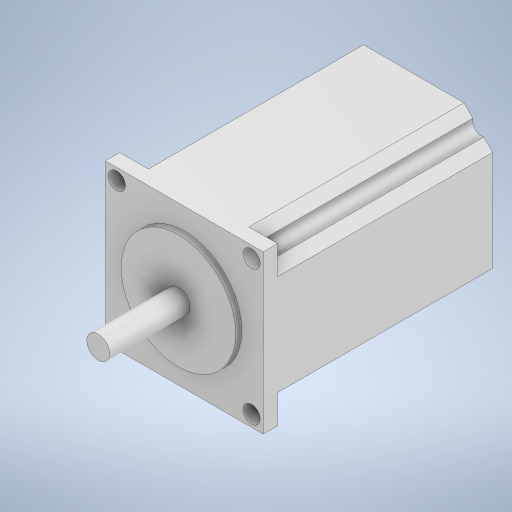
# Autodesk Inventor part: stepper motor base
Saved by Autodesk Inventor 2024 (Build 280153000, 153)
## iProperties
Created: 2023-10-26
Part Number: stepper motor base
Material: Aluminum
Document SubType Name: Modeling
Designer: mb
Density: 2.7 g/cm^3
Appearance: Satin
Author: mb
Autodesk Inventor part; units mm, degrees
ref_plane "YZ Plane" through (0, 0, 0) normal (1, 0, 0) x (0, 1, 0)
ref_plane "XZ Plane" through (0, 0, 0) normal (0, 1, 0) x (-1, 0, 0)
ref_plane "XY Plane" through (0, 0, 0) normal (0, 0, 1) x (1, 0, 0)
sketch "Sketch1" plane through (0, 0, 0) normal (0, 0, 1) x (1, 0, 0)
  line L0 (0, 0) -> (55, 0)
  line L1 (55, 0) -> (55, 55)
  line L2 (55, 55) -> (0, 55)
  line L3 (0, 55) -> (0, 0)
  dimension "d0" = 55
  dimension "d1" = 55
  constraints: 8 end point, 2 parallel, 1 horizontal, 1 perpendicular
  measures "d0" distance of L1.end L2.end
  measures "d1" distance of L0.end L1.end
extrude "Extrusion1" add sketch "Sketch1" along normal blind 80
sketch "Sketch2" plane through (0, 0, 80) normal (0, 0, 1) x (1, 0, 0)
  line L0 (55, 0) -> (55, 55) projected
  line L1 (55, 55) -> (0, 55) projected
  line L2 (0, 55) -> (0, 0) projected
  line L3 (0, 0) -> (55, 0) projected
  circle A0 centre (27.5, 27.5) radius 20
  circle A1 centre (27.5, 27.5) radius 4
  dimension "d7" = 27.5
  dimension "d8" = 27.5
  dimension "d9" = 40
  dimension "d10" = 8
  constraints: 2 centre point, 1 coincident
  measures "d7" distance from line of L1 A0.centre
  measures "d8" distance from line of L2 A0.centre
  measures "d9" diameter of A0
  measures "d10" diameter of A1
extrude "Extrusion2" add sketch "Sketch2" along normal blind 2 contours A0
sketch "Sketch3" plane through (27.5, 27.5, 80) normal (0, 0, 1) x (1, 0, 0)
  circle A0 centre (0, 0) radius 4 projected
  point P0 (-27.5, -27.5)
extrude "Extrusion3" add sketch "Sketch3" along normal blind 30
chamfer "Chamfer1" distance 10 angle 45 4 edges at (0, 55, 40) (0, 0, 40) (55, 0, 40) (55, 55, 40)
sketch "Sketch4" plane through (0, 0, 80) normal (0, 0, 1) x (1, 0, 0)
  line L0 (45, 55) -> (55, 45) projected
  line L1 (45, 55) -> (10, 55) projected
  line L2 (0, 45) -> (10, 55) projected
  line L3 (0, 45) -> (0, 10) projected
  line L4 (10, 0) -> (0, 10) projected
  line L5 (10, 0) -> (45, 0) projected
  line L6 (55, 10) -> (45, 0) projected
  line L7 (55, 10) -> (55, 45) projected
  circle A0 centre (27.5, 27.5) radius 20 projected
  line L8 (10, 55) -> (0, 55)
  line L9 (0, 55) -> (0, 45)
  line L10 (0, 10) -> (0, 0)
  line L11 (0, 0) -> (10, 0)
  line L12 (45, 0) -> (55, 0)
  line L13 (55, 0) -> (55, 10)
  line L14 (55, 45) -> (55, 55)
  line L15 (45, 55) -> (55, 55)
  constraints: 16 end point, 4 perpendicular, 4 point on line, 1 horizontal, 1 vertical
extrude "Extrusion4" add sketch "Sketch4" against normal blind 5 contours L15 L14 L0 | L2 L9 L8 | L13 L12 L6 | L4 L11 L10
sketch "Sketch5" plane through (0, 0, 80) normal (0, 0, 1) x (1, 0, 0)
  line L0 (0, 45) -> (10, 55) projected
  circle A0 centre (4, 51) radius 3
  line L1 (55, 55) -> (0, 55) projected
  line L2 (0, 55) -> (0, 0) projected
  circle A1 centre (4, 4) radius 3
  circle A2 centre (51, 4) radius 3
  circle A3 centre (51, 51) radius 3
  line L3 (0, 0) -> (55, 0) projected
  line L4 (55, 0) -> (55, 55) projected
  dimension "d20" = 4
  dimension "d21" = 4
  dimension "d22" = 6
  dimension "d23" = 4
  dimension "d24" = 4
  dimension "d25" = 4
  dimension "d26" = 4
  dimension "d27" = 4
  dimension "d28" = 4
  constraints: 4 centre point, 3 equal radius
  measures "d20" distance from line of L1 A0.centre
  measures "d21" distance from line of L2 A0.centre
  measures "d22" diameter of A0
  measures "d23" distance from line of L3 A1.centre
  measures "d24" distance from line of L2 A1.centre
  measures "d25" distance from line of L3 A2.centre
  measures "d26" distance from line of L4 A2.centre
  measures "d27" distance from line of L4 A3.centre
  measures "d28" distance from line of L1 A3.centre
extrude "Extrusion5" cut sketch "Sketch5" against normal through all contours A0 L0 | L0 A0 | A1 | A2 | A3
equation "\"d7\" = 0.5 * d1"
equation "\"d8\" = 0.5 * d0"
body "Solid1"
